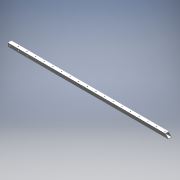
# Autodesk Inventor part: Main Extrusions
Saved by Autodesk Inventor 2019.4 (Build 234330000, 330)
## iProperties
Created: 2020-01-18
Part Number: Main Extrusions
Material: Aluminum 6061
Document SubType Name: Modeling
Designer: Mark
Mass: 348.459 g
Surface Area: 1318.95 cm^2
Volume: 129.059 cm^3
Density: 2.7 g/cm^3
Appearance: Aluminum - Flat
Author: Mark
Autodesk Inventor part; units mm, degrees
ref_plane "YZ Plane" through (0, 0, 0) normal (1, 0, 0) x (0, 1, 0)
ref_plane "XZ Plane" through (0, 0, 0) normal (0, 1, 0) x (-1, 0, 0)
ref_plane "XY Plane" through (0, 0, 0) normal (0, 0, 1) x (1, 0, 0)
sketch "Sketch1" plane through (0, 0, 0) normal (1, 0, 0) x (0, 1, 0)
  line L0 (-10, 10) -> (10, 10)
  line L1 (10, 10) -> (10, -10)
  line L2 (10, -10) -> (-10, -10)
  line L3 (-10, -10) -> (-10, 10)
  line L4 (-10, 10) -> (10, -10) construction
  line L5 (10, 10) -> (-10, -10) construction
  line L6 (-8, 8) -> (8, 8)
  line L7 (8, 8) -> (8, -8)
  line L8 (8, -8) -> (-8, -8)
  line L9 (-8, -8) -> (-8, 8)
  line L10 (-8, 8) -> (8, -8) construction
  line L11 (8, 8) -> (-8, -8) construction
  point P0 (0, 0)
  dimension "d0" = 20
  dimension "d1" = 20
  dimension "d2" = 16
  dimension "d3" = 16
  constraints: 24 end point, 4 midpoint, 4 parallel, 2 horizontal, 2 perpendicular
  measures "d0" distance of L1.end L2.end
  measures "d1" distance of L0.end L1.end
  measures "d2" distance of L7.end L8.end
  measures "d3" distance of L6.end L7.end
extrude "Extrusion1" add sketch "Sketch1" along normal blind 930
sketch "Sketch2" plane through (0, -10, -10) normal (0, 0, -1) x (-1, 0, 0)
  line L0 (-930, 0) -> (-930, 20) projected
  line L1 (-930, 0) -> (-910, 20)
  line L2 (0, 20) -> (-930, 20) projected
  point P0 (0, 10)
  dimension "d6" = 20
  constraints: 2 end point, 1 point on line
  measures "d6" distance from line of L0 L1.end
extrude "Extrusion2" cut sketch "Sketch2" against normal blind 20
sketch "Sketch3" plane through (0, 10, 10) normal (0, 1, 0) x (1, 0, 0)
  circle A0 centre (50, 10) radius 2.75
  line L0 (0, 20) -> (910, 20) projected
  line L1 (0, 0) -> (0, 20) projected
  circle A1 centre (100, 10) radius 2.75
  circle A2 centre (150, 10) radius 2.75
  circle A3 centre (200, 10) radius 2.75
  circle A4 centre (250, 10) radius 2.75
  circle A5 centre (300, 10) radius 2.75
  circle A6 centre (350, 10) radius 2.75
  circle A7 centre (400, 10) radius 2.75
  circle A8 centre (450, 10) radius 2.75
  circle A9 centre (500, 10) radius 2.75
  circle A10 centre (550, 10) radius 2.75
  circle A11 centre (600, 10) radius 2.75
  circle A12 centre (650, 10) radius 2.75
  circle A13 centre (700, 10) radius 2.75
  circle A14 centre (750, 10) radius 2.75
  circle A15 centre (800, 10) radius 2.75
  circle A16 centre (850, 10) radius 2.75
  circle A17 centre (900, 10) radius 2.75
  circle A18 centre (950, 10) radius 2.75
  circle A19 centre (1000, 10) radius 2.75
  point P0 (0, 10)
  dimension "d9" = 5.5
  dimension "d10" = 10
  dimension "d11" = 50
  dimension "d14" = 50
  constraints: 20 centre point, 1 horizontal, 38 other
  measures "d9" diameter of A0
  measures "d10" distance from line of L0 A0.centre
  measures "d11" distance from line of L1 A0.centre
  measures "d14" distance of A0.centre A1.centre
extrude "Extrusion3" cut sketch "Sketch3" against normal blind 20 contours A0 | A1 | A2 | A3 | A4 | A5 | A6 | A7 | A8 | A9 | A10 | A11 | A12 | A13 | A14 | A15 | A16 | A17
sketch "Sketch4" plane through (0, -10, 10) normal (0, 0, 1) x (1, 0, 0)
  circle A0 centre (10, 10) radius 2.75
  line L0 (0, 0) -> (930, 0) projected
  line L1 (0, 0) -> (0, 20) projected
  circle A1 centre (60, 10) radius 2.75
  circle A2 centre (110, 10) radius 2.75
  circle A3 centre (160, 10) radius 2.75
  circle A4 centre (210, 10) radius 2.75
  circle A5 centre (260, 10) radius 2.75
  circle A6 centre (310, 10) radius 2.75
  circle A7 centre (360, 10) radius 2.75
  circle A8 centre (410, 10) radius 2.75
  circle A9 centre (460, 10) radius 2.75
  circle A10 centre (510, 10) radius 2.75
  circle A11 centre (560, 10) radius 2.75
  circle A12 centre (610, 10) radius 2.75
  circle A13 centre (660, 10) radius 2.75
  circle A14 centre (710, 10) radius 2.75
  circle A15 centre (760, 10) radius 2.75
  circle A16 centre (810, 10) radius 2.75
  circle A17 centre (860, 10) radius 2.75
  circle A18 centre (910, 10) radius 2.75
  circle A19 centre (960, 10) radius 2.75
  point P0 (0, 10)
  dimension "d21" = 5.5
  dimension "d22" = 10
  dimension "d23" = 10
  dimension "d26" = 50
  constraints: 20 centre point, 1 horizontal, 38 other
  measures "d21" diameter of A0
  measures "d22" distance from line of L0 A0.centre
  measures "d23" distance from line of L1 A0.centre
  measures "d26" distance of A0.centre A1.centre
extrude "Extrusion4" cut sketch "Sketch4" against normal blind 20 contours A0 | A1 | A2
body "Solid1"
